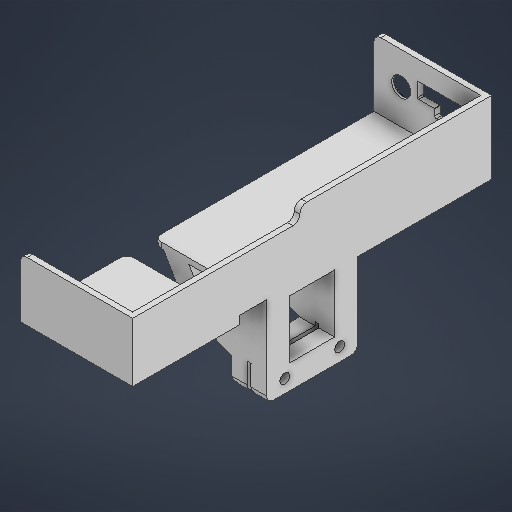
# Autodesk Inventor part: Copy of Revised Battery and Rotation Sensor Holder
Saved by Autodesk Inventor 2025.1 (Build 291241020, 241B)
## iProperties
Created: 2024-12-11
Part Number: Copy of Revised Battery and Rotation Sensor Holder
Material: Generic
Document SubType Name: Modeling
Designer: AtuStem
Density: 1 g/cm^3
Appearance: Default
Author: AtuStem
Autodesk Inventor part; units mm, degrees
ref_plane "YZ Plane" through (0, 0, 0) normal (1, 0, 0) x (0, 1, 0)
ref_plane "XZ Plane" through (0, 0, 0) normal (0, 1, 0) x (-1, 0, 0)
ref_plane "XY Plane" through (0, 0, 0) normal (0, 0, 1) x (1, 0, 0)
sketch "Sketch1" plane through (0, 0, 0) normal (1, 0, 0) x (0, 1, 0)
  line L0 (0, 0) -> (0, -12.7)
  circle A0 centre (0, -12.7) radius 3.9624
  line L1 (-6.096, -21.0566) -> (5.08, -21.0566)
  line L2 (5.08, -21.0566) -> (5.08, 0.0254)
  line L3 (5.08, 0.0254) -> (-6.096, 0.0254)
  line L4 (-6.096, 0.0254) -> (-6.096, -21.0566)
  line L5 (5.08, -10.3378) -> (34.544, -10.3378)
  line L6 (34.544, -10.3378) -> (34.544, -21.0566)
  line L7 (34.544, -21.0566) -> (5.08, -21.0566)
  line L8 (5.08, -21.0566) -> (5.08, -10.3378)
  line L9 (34.544, -83.1596) -> (32.004, -83.1596)
  line L10 (32.004, -83.1596) -> (32.004, 83.2104)
  line L11 (34.544, 83.2104) -> (34.544, -83.1596)
  line L12 (0, 0) -> (0, 12.7508)
  circle A1 centre (0, 12.7508) radius 3.9624
  line L13 (-6.096, 21.1074) -> (5.08, 21.1074)
  line L14 (5.08, 21.1074) -> (5.08, 0.0254)
  line L15 (-6.096, 0.0254) -> (-6.096, 21.1074)
  line L16 (5.08, 10.3886) -> (34.544, 10.3886)
  line L17 (34.544, 10.3886) -> (34.544, 21.1074)
  line L18 (34.544, 21.1074) -> (5.08, 21.1074)
  line L19 (5.08, 21.1074) -> (5.08, 10.3886)
  line L20 (34.544, 83.2104) -> (32.004, 83.2104)
  circle A2 centre (0, -12.7) radius 2.286
  circle A3 centre (0, 12.7508) radius 2.286
  point P0 (5.08, -21.0566)
  point P1 (32.004, -21.0566)
  point P2 (32.004, -10.3378)
  point P3 (33.274, -83.1596)
  point P4 (34.544, -21.0566)
  point P5 (32.004, 21.1074)
  point P6 (34.544, 21.1074)
  point P7 (32.004, 10.3886)
  point P8 (34.544, 10.3886)
  point P9 (34.544, -10.3378)
  point P10 (5.08, 21.1074)
  dimension "d0" = 12.7
  dimension "d1" = 7.9248
  dimension "d3" = 6.096
  dimension "d4" = 5.08
  dimension "d8" = 10.3632
  dimension "d9" = 29.464
  dimension "d11" = 2.54
  dimension "d32" = 4.572
  dimension "d34" = 4.572
  dimension "d96" = 26.924
  dimension "d117" = 8.3566
  dimension "d120" = 166.37
  dimension "d145" = 10.7188
  dimension "d146" = 10.7188
  dimension "d149" = 0
  constraints: 42 end point, 10 symmetric about line, 5 parallel, 4 centre point, 4 coincident, 3 horizontal, 3 perpendicular, 2 point on line, 1 midpoint, 1 vertical, 1 other
  measures "d0" distance of L0.start L0.end
  measures "d1" diameter of A0
  measures "d3" distance from line of L4 L0.end
  measures "d4" distance from line of L2 L0.end
  measures "d8" distance between parallel lines of L3 L5
  measures "d9" distance of L5.start L5.end
  measures "d11" distance of L9.start L9.end
  measures "d32" diameter of A3
  measures "d34" diameter of A2
  measures "d96" distance between parallel lines of L8 L10
  measures "d117" distance from line of L1 A2.centre
  measures "d120" distance between parallel lines of L20 L9
  measures "d145" distance between parallel lines of L5 L7
  measures "d146" distance between parallel lines of L18 L16
  measures "d149" distance between parallel lines of L1 L7
extrude "Extrusion1" add sketch "Sketch1" along normal blind 16.2306 contours A0 | L4 L3 L2 L1 | L2 L5 L10 L7 | L15 L13 L14 L3 | L2 L14 L16 L10 L5 | L10 L5 L6 L7 | L7 L11 L9 L10 | L18 L10 L16 L14 | L10 L18 L11 L16 | L10 L20 L11 L18 | A1 | A2 | A3
extrude "Extrusion2" add sketch "Sketch1" along normal blind 16.2306 and the other way blind 35.814 contours L10 L5 L6 L7 | L7 L11 L9 L10 | L10 L16 L11 L5 | L10 L18 L11 L16 | L10 L20 L11 L18
extrude "Extrusion3" cut sketch "Sketch1" along normal blind 2.54 contours A0 | A1 | A2 | A3
extrude "Extrusion4" cut sketch "Sketch1" along normal up to surface (16.2306 mm away) contours A2 | A3
sketch "Sketch3" plane through (0, -6.096, 21.1074) normal (0, 0, 1) x (1, 0, 0)
  line L0 (0, 0) -> (16.2306, 0) projected
  line L1 (7.2644, 0) -> (8.9662, 0)
  line L2 (8.9662, 0) -> (8.9662, 12.7)
  line L3 (8.9662, 12.7) -> (7.2644, 12.7)
  line L4 (7.2644, 12.7) -> (7.2644, 0)
  line L5 (16.2306, 38.1) -> (16.2306, 0) projected
  line L6 (0, 38.1) -> (0, 0) projected
  point P0 (0, 6.096)
  point P1 (16.2306, 11.176)
  point P2 (0, 11.176)
  dimension "d37" = 1.7018
  dimension "d38" = 12.7
  dimension "d39" = 16.2306
  dimension "d40" = 7.2644
  dimension "d41" = 7.2644
  constraints: 8 end point, 2 parallel, 1 horizontal, 1 perpendicular, 1 point on line
  measures "d37" distance between parallel lines of L2 L4
  measures "d38" distance of L1.end L2.end
  measures "d39" distance between parallel lines of L5 L6
  measures "d40" distance between parallel lines of L5 L2
  measures "d41" distance between parallel lines of L4 L6
extrude "Extrusion5" cut sketch "Sketch3" against normal up to surface (42.164 mm away)
sketch "Sketch13" plane through (16.2306, 0, 0) normal (1, 0, 0) x (0, 0, -1)
  line L0 (-10.3505, 5.08) -> (-10.3505, 32.004) projected
  line L1 (10.3505, 5.08) -> (-10.3505, 5.08) projected
  line L2 (-10.3505, 32.004) -> (10.3505, 32.004)
  line L3 (10.3505, 32.004) -> (10.3505, 5.08)
  line L4 (10.3505, 5.08) -> (-10.3505, 5.08)
  line L5 (-10.3505, 5.08) -> (-10.3505, 32.004)
  point P0 (0, 0)
  point P1 (-10.3505, 16.0828)
  constraints: 8 end point, 2 parallel, 1 horizontal, 1 perpendicular
extrude "Extrusion14" cut sketch "Sketch13" against normal blind 63.5
sketch "Sketch16" plane through (16.2306, 5.08, -10.3505) normal (0, 0, 1) x (1, 0, 0)
  line L0 (-16.2306, 34.29) -> (-33.7312, 34.29)
  line L1 (-33.7312, 34.29) -> (-33.7312, 0)
  line L2 (-33.7312, 0) -> (-16.2306, 0)
  line L3 (-16.2306, 0) -> (-16.2306, 34.29)
  line L4 (-16.2306, 0) -> (-33.7312, 0)
  line L5 (-33.7312, 0) -> (-33.7312, 12.7762)
  line L6 (-16.2306, 12.7762) -> (-16.2306, 0)
  circle A0 centre (-33.7312, 12.7762) radius 5.08
  circle A1 centre (-33.7312, 12.7762) radius 2.286
  line L7 (-16.2306, 0) -> (-35.6811, 8.0853)
  line L8 (-31.7813, 17.4671) -> (-16.2306, 11.0028)
  line L9 (-33.7312, 34.29) -> (-51.988, 34.29)
  line L10 (-52.0446, 34.29) -> (-38.1285, 10.2326)
  line L11 (-29.3339, 15.3198) -> (-40.3072, 34.29)
  line L12 (-16.2306, 0) -> (-16.2306, 2.7259)
  line L13 (-16.2306, 0) -> (-16.2306, 26.924) projected
  line L14 (-47.7837, 26.924) -> (-36.0464, 26.924)
  line L15 (-16.2306, 26.924) -> (-91.44, 26.924) projected
  point P0 (-16.2306, -5.08)
  point P1 (-37.0181, 16.6495)
  point P2 (-30.1944, 16.8074)
  dimension "d132" = 17.5006
  dimension "d133" = 10.16
  dimension "d134" = 4.572
  constraints: 28 end point, 6 point on line, 5 point on circle, 3 parallel, 3 tangent, 2 centre point, 2 coincident, 2 horizontal, 2 perpendicular
  measures "d132" distance between parallel lines of L1 L3
  measures "d133" diameter of A0
  measures "d134" diameter of A1
extrude "Extrusion17" add sketch "Sketch16" along normal up to surface (31.4579 mm away) contours L11 L8 A0 L1 | L1 A0 L10 L14 L11 | L3 L7 L1 A0 L11 L8 | A0 L1 A1 | L1 A1 A0 | L11 A0 L8 | A0 L1 L7
sketch "Sketch17" plane through (16.2306, 0, 0) normal (1, 0, 0) x (0, 0, -1)
  line L0 (-10.3505, 32.004) -> (-21.1074, 32.004) projected
  line L1 (10.3505, 6.604) -> (10.3505, 5.08) projected
  line L2 (-10.3505, 32.004) -> (10.3505, 32.004)
  line L3 (10.3505, 32.004) -> (10.3505, 5.08)
  line L4 (10.3505, 5.08) -> (-10.3505, 5.08)
  line L5 (-10.3505, 5.08) -> (-10.3505, 32.004)
  point P0 (0, 0)
  point P1 (-19.6723, 32.004)
  constraints: 8 end point, 2 parallel, 1 horizontal, 1 perpendicular
extrude "Extrusion18" cut sketch "Sketch17" against normal blind 101.6
fillet "Fillet18" radius 3.175 1 edges at (-13.9638, 21.8874, 15.729)
fillet "Fillet19" radius 3.175 5 edges at (0, -6.096, 0.0254) (3.6322, -6.096, -21.0566) (12.5984, -6.096, -21.0566) (3.6322, -6.096, 21.1074) (12.5984, -6.096, 21.1074)
extrude "Extrusion19" add sketch "Sketch16" against normal up to surface (10.7061 mm away) contours L11 L8 A0 L1 | L1 A0 L10 L14 L11 | L3 L7 L1 A0 L11 L8 | A0 L1 A1 | L1 A1 A0 | L11 A0 L8 | A0 L1 L7
sketch "Sketch18" plane through (16.2306, 34.544, 83.2104) normal (0, 1, 0) x (1, 0, 0)
  line L0 (-52.0446, 166.37) -> (0, 166.37) projected
  line L1 (-52.0446, 0) -> (0, 0) projected
  line L2 (-52.0446, 166.37) -> (-49.7211, 166.37)
  line L3 (-49.7211, 166.37) -> (-49.7211, 0)
  line L4 (-49.7211, 0) -> (-52.0446, 0)
  line L5 (-52.0446, 0) -> (-52.0446, 166.37)
  line L6 (0, 0) -> (-2.54, 0)
  line L7 (-2.54, 0) -> (-2.54, 166.37)
  line L8 (-2.54, 166.37) -> (0, 166.37)
  line L9 (0, 166.37) -> (0, 0)
  line L10 (-52.0446, 163.83) -> (0, 163.83)
  line L11 (0, 163.83) -> (0, 166.37)
  line L12 (0, 166.37) -> (-52.0446, 166.37)
  line L13 (-52.0446, 166.37) -> (-52.0446, 163.83)
  line L14 (-52.0446, 0) -> (0, 0)
  line L15 (0, 0) -> (0, 2.54)
  line L16 (0, 2.54) -> (-52.0446, 2.54)
  line L17 (-52.0446, 2.54) -> (-52.0446, 0)
  line L18 (-2.54, 77.47) -> (0, 77.47)
  line L19 (0, 77.47) -> (0, 0)
  line L20 (0, 0) -> (-2.54, 0)
  line L21 (-2.54, 0) -> (-2.54, 77.47)
  point P0 (-16.2306, 83.2104)
  point P1 (0, 166.37)
  point P2 (-2.54, 163.83)
  point P3 (-2.54, 2.54)
  point P4 (-52.0446, 2.54)
  dimension "d153" = 2.54
  dimension "d154" = 2.54
  dimension "d155" = 2.54
  dimension "d164" = 88.9
  constraints: 40 end point, 10 parallel, 5 horizontal, 5 perpendicular, 5 point on line
  measures "d153" distance between parallel lines of L10 L0
  measures "d154" distance between parallel lines of L9 L7
  measures "d155" distance between parallel lines of L1 L16
  measures "d164" distance between parallel lines of L18 L0
extrude "Extrusion20" add sketch "Sketch18" along normal blind 31.115 contours L0 L3 L10 L5 | L0 L7 L10 L3 | L0 L9 L10 L7 | L16 L3 L1 L5 | L10 L9 L18 L7 | L16 L7 L1 L3 | L18 L9 L16 L7 | L16 L9 L1 L7
sketch "Sketch19" plane through (16.2306, 32.004, -83.1596) normal (0, 0, -1) x (-1, 0, 0)
  line L0 (7.9478, 18.1985) -> (7.9478, 24.3407)
  line L1 (8.4478, 24.8408) -> (31.2478, 24.8408)
  line L2 (23.1678, 13.9371) -> (16.5278, 13.9371)
  line L3 (15.6762, 17.6984) -> (8.4478, 17.6984)
  line L4 (31.2478, 17.6984) -> (24.0194, 17.6984)
  line L5 (31.7478, 24.3407) -> (31.7478, 18.1985)
  line L6 (15.7778, 14.6873) -> (15.7778, 17.5968)
  line L7 (23.9178, 17.5968) -> (23.9178, 14.6873)
  ellipse E0 centre (16.5278, 14.6873) end of major axis (16.5278, 13.9371) minor radius 0.75 (15.7778, 14.6873) -> (16.5278, 13.9371) ccw
  ellipse E1 centre (23.1678, 14.6873) end of major axis (23.1678, 13.9371) minor radius 0.75 (23.1678, 13.9371) -> (23.9178, 14.6873) ccw
  arc A0 (15.7778, 17.5968) -> (15.6762, 17.6984) centre (15.6762, 17.5968) ccw
  arc A1 (24.0194, 17.6984) -> (23.9178, 17.5968) centre (24.0194, 17.5968) ccw
  ellipse E2 centre (8.4478, 18.1985) end of major axis (8.4478, 17.6984) minor radius 0.5 (7.9478, 18.1985) -> (8.4478, 17.6984) ccw
  ellipse E3 centre (8.4478, 24.3407) end of major axis (8.4478, 23.8405) minor radius 0.5 (8.4478, 24.8408) -> (7.9478, 24.3407) ccw
  ellipse E4 centre (31.2478, 24.3407) end of major axis (31.2478, 23.8405) minor radius 0.5 (31.7478, 24.3407) -> (31.2478, 24.8408) ccw
  ellipse E5 centre (31.2478, 18.1985) end of major axis (31.2478, 17.6984) minor radius 0.5 (31.2478, 17.6984) -> (31.7478, 18.1985) ccw
  circle A2 centre (39.4178, 18.6639) radius 6.0325
  circle A3 centre (39.4178, 18.6639) radius 4.445
  line L8 (0, 6.35) -> (0, 33.655)
  line L9 (0, 33.655) -> (52.0446, 33.655)
  line L10 (52.0446, 6.35) -> (52.0446, 33.655)
  line L11 (45.6946, 0) -> (6.35, 0)
  arc A4 (0, 6.35) -> (6.35, 0) centre (6.35, 6.35) ccw
  arc A5 (45.6946, 0) -> (52.0446, 6.35) centre (45.6946, 6.35) ccw
  line L12 (0, 33.655) -> (52.0446, 33.655) projected
  line L13 (0, 0) -> (0, 33.655) projected
  point P0 (16.2306, -32.004)
  constraints: 24 end point, 8 point on circle, 6 centre point, 24 other
extrude "Extrusion21" cut sketch "Sketch19" against normal up to surface (2.54 mm away) contours L0 E3 L1 E4 L5 E5 L4 A1 L7 E1 L2 E0 L6 A0 L3 E2 | A3
chamfer "Chamfer3" distance 1.5875 angle 45 1 edges at (-18.7422, 50.6679, -83.1596)
sketch "Sketch20" plane through (16.2306, 0, 0) normal (1, 0, 0) x (0, 0, -1)
  line L0 (-83.2104, 32.004) -> (-83.2104, 65.659) projected
  line L1 (-83.2104, 65.659) -> (-5.7404, 65.659)
  line L2 (-5.7404, 65.659) -> (-5.7404, 59.3598)
  line L3 (-5.7404, 59.3598) -> (-83.2104, 59.3598)
  line L4 (-83.2104, 59.3598) -> (-83.2104, 65.659)
  line L5 (83.1596, 32.004) -> (83.1596, 65.659) projected
  point P0 (0, 0)
  dimension "d165" = 88.9
  dimension "d166" = 6.2992
  constraints: 8 end point, 2 parallel, 1 horizontal, 1 perpendicular
  measures "d165" distance between parallel lines of L2 L5
  measures "d166" distance between parallel lines of L1 L3
extrude "Extrusion22" cut sketch "Sketch20" against normal up to surface (52.0446 mm away)
fillet "Fillet23" radius 3.175 1 edges at (14.9606, 65.659, 5.7404)
fillet "Fillet24" radius 3.175 3 edges at (-35.814, 59.3598, 81.9404) (-35.814, 65.659, -81.8896) (14.9606, 59.3598, 5.7404)
sketch "Sketch21" plane through (16.2306, 0, 0) normal (1, 0, 0) x (0, 0, -1)
  line L0 (-21.1074, 32.004) -> (-21.1074, -2.921) projected
  line L1 (-21.1074, 32.004) -> (-33.8074, 32.004)
  line L2 (-33.8074, 32.004) -> (-33.8074, 35.814)
  line L3 (-33.8074, 35.814) -> (-21.1074, 35.814)
  line L4 (-21.1074, 35.814) -> (-21.1074, 32.004)
  point P0 (0, 0)
  point P1 (21.0566, 32.004)
  dimension "d171" = 12.7
  dimension "d173" = 3.81
  constraints: 8 end point, 2 parallel, 1 horizontal, 1 perpendicular
  measures "d171" distance between parallel lines of L4 L2
  measures "d173" distance between parallel lines of L1 L3
fillet "Fillet26" radius 6.35 1 edges at (13.6906, 34.544, 0.0254)
extrude "Extrusion24" cut sketch "Sketch21" against normal up to surface (52.0446 mm away)
fillet "Fillet27" radius 3.175 2 edges at (-35.814, 33.274, 21.1074) (-35.814, 33.274, 33.8074)
body "Solid1"
